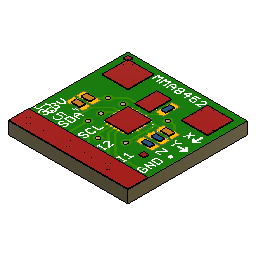
Potted Sensor v16 (Autodesk Fusion 360 archive; units mm, degrees)
design "SparkFun_MMA8452Q-Breakout"
part number: MMA8452Q
part number: 4.7uF
part number: 10k
part number: OSHW-LOGOS
part number: LOGO-SFESK
part number: STAND-OFF
part number: FIDUCIALUFIDUCIAL
Autodesk Fusion 360 part; units mm, degrees
sketch "sketch 306" plane through (0, 0, 0) normal (0, 0, 1) x (1, 0, 0)
  line L0 (0, 0) -> (0, 15.24)
  line L1 (0, 15.24) -> (15.24, 15.24)
  line L2 (15.24, 15.24) -> (15.24, 0)
  line L3 (15.24, 0) -> (0, 0)
extrude "Board" add sketch "sketch 306" along normal blind 1.57 makes body 1 in component "Board"
sketch "sketch 618" plane through (0, 0, 0) normal (0, 0, 1) x (1, 0, 0)
  line L0 (-1.5, -1.5) -> (1.5, -1.5)
  line L1 (1.5, -1.5) -> (1.5, 1.5)
  line L2 (1.5, 1.5) -> (-1.5, 1.5)
  line L3 (-1.5, 1.5) -> (-1.5, -1.5)
extrude "QFN-16_0.5MM" add sketch "sketch 618" along normal blind 0.1 separate body makes body 2 in component "QFN-16_0.5MM"
sketch "sketch 769" plane through (0, 0, 0) normal (0, 0, 1) x (1, 0, 0)
  line L0 (-0.554, -0.305) -> (0.559, -0.305)
  line L1 (0.559, -0.305) -> (0.559, 0.295)
  line L2 (0.559, 0.295) -> (-0.554, 0.295)
  line L3 (-0.554, 0.295) -> (-0.554, -0.305)
extrude "0402-CAP" add sketch "sketch 769" along normal blind 0.1 separate body makes body 3 in component "0402-CAP"
sketch "sketch 920" plane through (0, 0, 0) normal (0, 0, 1) x (1, 0, 0)
  line L0 (-0.554, -0.356) -> (0.559, -0.356)
  line L1 (0.559, -0.356) -> (0.559, 0.356)
  line L2 (0.559, 0.356) -> (-0.554, 0.356)
  line L3 (-0.554, 0.356) -> (-0.554, -0.356)
extrude "0402-RES" add sketch "sketch 920" along normal blind 0.1 separate body makes body 4 in component "0402-RES"
sketch "sketch 1055" plane through (0, 0, 0) normal (0, 0, 1) x (1, 0, 0)
  line L0 (-1.489, -1.182) -> (1.489, -1.182)
  line L1 (1.489, -1.182) -> (1.489, 1.489)
  line L2 (1.489, 1.489) -> (-1.489, 1.489)
  line L3 (-1.489, 1.489) -> (-1.489, -1.182)
extrude "OSHW-LOGO-S" add sketch "sketch 1055" along normal blind 0.1 separate body makes body 5 in component "OSHW-LOGO-S"
sketch "sketch 1190" plane through (0, 0, 0) normal (0, 0, 1) x (1, 0, 0)
  line L0 (0, 0.002) -> (1.859, 0.002)
  line L1 (1.859, 0.002) -> (1.859, 2.804)
  line L2 (1.859, 2.804) -> (0, 2.804)
  line L3 (0, 2.804) -> (0, 0.002)
extrude "SFE-LOGO-FLAME" add sketch "sketch 1190" along normal blind 0.1 separate body makes body 6 in component "SFE-LOGO-FLAME"
sketch "sketch 1333" plane through (0, 0, 0) normal (0, 0, 1) x (1, 0, 0)
  line L0 (-1.651, -1.651) -> (1.651, -1.651)
  line L1 (1.651, -1.651) -> (1.651, 1.651)
  line L2 (1.651, 1.651) -> (-1.651, 1.651)
  line L3 (-1.651, 1.651) -> (-1.651, -1.651)
extrude "STAND-OFF" add sketch "sketch 1333" along normal blind 0.1 separate body makes body 7 in component "STAND-OFF"
sketch "sketch 1468" plane through (0, 0, 0) normal (0, 0, 1) x (1, 0, 0)
  line L0 (-1.27, -1.27) -> (13.97, -1.27)
  line L1 (13.97, -1.27) -> (13.97, 1.27)
  line L2 (13.97, 1.27) -> (-1.27, 1.27)
  line L3 (-1.27, 1.27) -> (-1.27, -1.27)
extrude "1X06" add sketch "sketch 1468" along normal blind 0.1 separate body makes body 8 in component "1X06"
sketch "sketch 1603" plane through (0, 0, 0) normal (0, 0, 1) x (1, 0, 0)
  line L0 (-1, -1) -> (1, -1)
  line L1 (1, -1) -> (1, 1)
  line L2 (1, 1) -> (-1, 1)
  line L3 (-1, 1) -> (-1, -1)
extrude "SJ_2S-NO" add sketch "sketch 1603" along normal blind 0.1 separate body makes body 9 in component "SJ_2S-NO"
sketch "sketch 1746" plane through (0, 0, 0) normal (0, 0, 1) x (1, 0, 0)
  line L0 (-0.3175, -0.3175) -> (0.3175, -0.3175)
  line L1 (0.3175, -0.3175) -> (0.3175, 0.3175)
  line L2 (0.3175, 0.3175) -> (-0.3175, 0.3175)
  line L3 (-0.3175, 0.3175) -> (-0.3175, -0.3175)
extrude "MICRO-FIDUCIAL" add sketch "sketch 1746" along normal blind 0.1 separate body makes body 10 in component "MICRO-FIDUCIAL"
sketch "sketch 413" plane through (0, 0, 0) normal (0, 0, 1) x (1, 0, 0)
  circle A0 centre (9.898, 5.08) radius 0.254
  circle A1 centre (5.461, 9.144) radius 0.254
  circle A2 centre (7.62, 3.81) radius 0.254
  circle A3 centre (3.81, 8.89) radius 0.254
  circle A4 centre (5.08, 5.08) radius 0.254
  circle A5 centre (5.08, 6.731) radius 0.254
  circle A6 centre (10.16, 10.16) radius 0.254
  circle A7 centre (2.54, 12.7) radius 1.651
  circle A8 centre (12.7, 12.7) radius 1.651
  circle A9 centre (1.27, 1.27) radius 0.508
  circle A10 centre (3.81, 1.27) radius 0.508
  circle A11 centre (6.35, 1.27) radius 0.508
  circle A12 centre (8.89, 1.27) radius 0.508
  circle A13 centre (11.43, 1.27) radius 0.508
  circle A14 centre (13.97, 1.27) radius 0.508
extrude "Extrude2" cut sketch "sketch 413" along normal blind 1.57 bodies 1 in component "Board"
component "PCB Component" placed x (1, 0, 0) y (0, 1, 0) z (0, 0, 1) at (0, 0, 0)
component "Board" placed x (1, 0, 0) y (0, 1, 0) z (0, 0, 1) at (0, 0, 0) in component "PCB Component"
component "QFN-16_0.5MM" placed x (0, -1, 0) y (1, 0, 0) z (0, 0, 1) at (7.62, 7.62, 1.57) in component "PCB Component"
component "0402-CAP" placed x (1, 0, 0) y (0, 1, 0) z (0, 0, 1) at (11.43, 7.62, 1.57) in component "PCB Component"
component "0402-CAP" placed x (0, 1, 0) y (-1, 0, 0) z (0, 0, 1) at (8.89, 11.43, 1.57) in component "PCB Component"
component "0402-CAP" placed x (1, 0, 0) y (0, 1, 0) z (0, 0, 1) at (11.43, 6.35, 1.57) in component "PCB Component"
component "0402-RES" placed x (-1, 0, 0) y (0, -1, 0) z (0, 0, 1) at (2.54, 7.62, 1.57) in component "PCB Component"
component "0402-RES" placed x (-1, 0, 0) y (0, -1, 0) z (0, 0, 1) at (2.54, 6.35, 1.57) in component "PCB Component"
component "0402-RES" placed x (-1, 0, 0) y (0, -1, 0) z (0, 0, 1) at (11.43, 8.89, 1.57) in component "PCB Component"
component "OSHW-LOGO-S" placed x (-1, 0, 0) y (0, 1, 0) z (0, 0, -1) at (7.62, 11.811, 0) in component "PCB Component"
component "SFE-LOGO-FLAME" placed x (1, 0, 0) y (0, 1, 0) z (0, 0, 1) at (6.223, 9.906, 1.57) in component "PCB Component"
component "STAND-OFF" placed x (1, 0, 0) y (0, 1, 0) z (0, 0, 1) at (2.54, 12.7, 1.57) in component "PCB Component"
component "STAND-OFF" placed x (1, 0, 0) y (0, 1, 0) z (0, 0, 1) at (12.7, 12.7, 1.57) in component "PCB Component"
component "1X06" placed x (1, 0, 0) y (0, 1, 0) z (0, 0, 1) at (1.27, 1.27, 1.57) in component "PCB Component"
component "SJ_2S-NO" placed x (0, 1, 0) y (1, 0, 0) z (0, 0, -1) at (7.62, 7.62, 0) in component "PCB Component"
component "MICRO-FIDUCIAL" placed x (1, 0, 0) y (0, 1, 0) z (0, 0, 1) at (12.446, 4.826, 1.57) in component "PCB Component"
component "MICRO-FIDUCIAL" placed x (1, 0, 0) y (0, 1, 0) z (0, 0, 1) at (0.762, 14.478, 1.57) in component "PCB Component"
named bodies: "Board", "QFN-16_0.5MM", "0402-CAP", "0402-RES", "OSHW-LOGO-S", "SFE-LOGO-FLAME", "STAND-OFF", "1X06", "SJ_2S-NO", "MICRO-FIDUCIAL"
